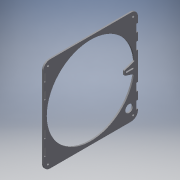
# Autodesk Inventor part: TrayPanelD_180mm
Saved by Autodesk Inventor 2017 (Build 210142000, 142)
## iProperties
Created: 2019-06-22
Part Number: TrayPanelD_180mm
Material: Generic
Document SubType Name: Modeling
Designer: DDeGo
Density: 1 g/cm^3
Appearance: Default
Author: DDeGo
Autodesk Inventor part; units mm, degrees
ref_plane "YZ Plane" through (0, 0, 0) normal (1, 0, 0) x (0, 1, 0)
ref_plane "XZ Plane" through (0, 0, 0) normal (0, 1, 0) x (-1, 0, 0)
ref_plane "XY Plane" through (0, 0, 0) normal (0, 0, 1) x (1, 0, 0)
sketch "Sketch1" plane through (0, 0, 0) normal (1, 0, 0) x (0, 1, 0)
  circle A0 centre (-4, -4) radius 2
  circle A1 centre (78.5, 78.5) radius 85
  circle A2 centre (161, -4) radius 2
  circle A3 centre (-4, 161) radius 2
  circle A4 centre (161, 161) radius 2
  line L0 (157, 170) -> (0, 170)
  arc A5 (0, 170) -> (-13, 157) centre (0, 157) ccw
  line L1 (-13, 157) -> (-13, 0)
  arc A6 (-13, 0) -> (0, -13) centre (0, 0) ccw
  line L2 (0, -13) -> (157, -13)
  arc A7 (157, -13) -> (170, 0) centre (157, 0) ccw
  line L3 (170, 0) -> (170, 157)
  arc A8 (170, 157) -> (157, 170) centre (157, 157) ccw
  line L4 (-4, 161) -> (161, 161) construction
  line L5 (161, 161) -> (161, -4) construction
  line L6 (161, -4) -> (-4, -4) construction
  line L7 (-4, -4) -> (-4, 161) construction
  line L8 (-4, 161) -> (161, -4) construction
  line L9 (-13, 78.5) -> (78.5, 78.5) construction
  line L10 (78.5, 78.5) -> (170, 78.5) construction
  dimension "d10" = 183
  dimension "d11" = 183
  dimension "d12" = 165
  dimension "d13" = 165
  dimension "d15" = 13
  dimension "d16" = 4
  dimension "d17" = 170
  constraints: 22 end point, 9 centre point, 8 point on circle, 8 tangent, 6 equal radius, 3 horizontal, 3 midpoint, 3 perpendicular, 1 coincident, 1 collinear, 1 vertical
  measures "d10" distance between parallel lines of L3 L1
  measures "d11" distance between parallel lines of L0 L2
  measures "d12" distance between parallel lines of L5 L7
  measures "d13" distance of L4.end L5.end
  measures "d15" radius of A5
  measures "d16" diameter of A4
  measures "d17" diameter of A1
extrude "Extrusion1" add sketch "Sketch1" along normal blind 2.75
sketch "Sketch2" plane through (2.75, 0, 0) normal (1, 0, 0) x (0, 0, -1)
  line L0 (0, 170) -> (-157, 170) projected
  line L1 (-146.1, 170) -> (-131.1, 170)
  line L2 (-131.1, 170) -> (-131.1, 166.5)
  line L3 (-131.1, 166.5) -> (-146.1, 166.5)
  line L4 (-146.1, 166.5) -> (-146.1, 170)
  line L5 (-116.1, 170) -> (-101.1, 170)
  line L6 (-101.1, 170) -> (-101.1, 166.5)
  line L7 (-101.1, 166.5) -> (-116.1, 166.5)
  line L8 (-116.1, 166.5) -> (-116.1, 170)
  line L9 (-47.1, 170) -> (-32.1, 170)
  line L10 (-32.1, 170) -> (-32.1, 166.5)
  line L11 (-32.1, 166.5) -> (-47.1, 166.5)
  line L12 (-47.1, 166.5) -> (-47.1, 170)
  line L13 (-2.1, 170) -> (-17.1, 170)
  line L14 (-17.1, 170) -> (-17.1, 166.5)
  line L15 (-17.1, 166.5) -> (-2.1, 166.5)
  line L16 (-2.1, 166.5) -> (-2.1, 170)
  circle A0 centre (-161, 161) radius 2 projected
  point P0 (0, 0)
  dimension "d2" = 15
  dimension "d3" = 30
  dimension "d4" = 69
  dimension "d5" = 30
  dimension "d6" = 3.5
  dimension "d7" = 14.9
  constraints: 32 end point, 8 parallel, 7 point on line, 4 horizontal, 4 perpendicular, 3 collinear
  measures "d2" distance of L2.end L3.end
  measures "d3" distance between parallel lines of L6 L2
  measures "d4" distance between parallel lines of L10 L6
  measures "d5" distance between parallel lines of L16 L10
  measures "d6" distance of L15.end L13.start
  measures "d7" distance from line of L4 A0.centre
extrude "Extrusion2" cut sketch "Sketch2" against normal blind 10 contours L16 L15 L14 L0 | L10 L11 L12 L0 | L6 L7 L8 L0 | L2 L3 L4 L0
sketch "Sketch3" plane through (2.75, 0, 0) normal (1, 0, 0) x (0, 0, -1)
  line L0 (-56.4, -11.425) -> (-41.4, -11.425)
  line L1 (-41.4, -11.425) -> (-41.4, -8.675)
  line L2 (-41.4, -8.675) -> (-56.4, -8.675)
  line L3 (-56.4, -8.675) -> (-56.4, -11.425)
  line L4 (-26.4, -11.425) -> (-11.4, -11.425)
  line L5 (-11.4, -11.425) -> (-11.4, -8.675)
  line L6 (-11.4, -8.675) -> (-26.4, -8.675)
  line L7 (-26.4, -8.675) -> (-26.4, -11.425)
  line L8 (-106.4, -11.425) -> (-121.4, -11.425)
  line L9 (-121.4, -11.425) -> (-121.4, -8.675)
  line L10 (-121.4, -8.675) -> (-106.4, -8.675)
  line L11 (-106.4, -8.675) -> (-106.4, -11.425)
  line L12 (-136.4, -11.425) -> (-151.4, -11.425)
  line L13 (-151.4, -11.425) -> (-151.4, -8.675)
  line L14 (-151.4, -8.675) -> (-136.4, -8.675)
  line L15 (-136.4, -8.675) -> (-136.4, -11.425)
  line L16 (-157, -13) -> (0, -13) projected
  circle A0 centre (-161, -4) radius 2 projected
  point P0 (0, 0)
  dimension "d18" = 1.575
  dimension "d19" = 30
  dimension "d20" = 65
  dimension "d21" = 30
  dimension "d22" = 2.75
  dimension "d23" = 9.6
  dimension "d26" = 15
  constraints: 32 end point, 8 parallel, 6 point on line, 4 horizontal, 4 perpendicular, 3 collinear
  measures "d18" distance between parallel lines of L16 L12
  measures "d19" distance between parallel lines of L11 L15
  measures "d20" distance between parallel lines of L1 L11
  measures "d21" distance between parallel lines of L5 L1
  measures "d22" distance of L4.end L5.end
  measures "d23" distance from line of A0.centre L13
  measures "d26" distance of L12.start L12.end
extrude "Extrusion3" cut sketch "Sketch3" against normal blind 10 contours L3 L2 L1 L0 | L7 L6 L5 L4 | L8 L9 L10 L11 | L12 L13 L14 L15
sketch "Sketch4" plane through (2.75, 0, 0) normal (1, 0, 0) x (0, 0, -1)
  line L0 (-75.85, 147) -> (-73.1, 147)
  line L1 (-73.1, 147) -> (-73.1, 162)
  line L2 (-73.1, 162) -> (-75.85, 162)
  line L3 (-75.85, 162) -> (-75.85, 147)
  line L4 (-78.85, 144) -> (-70.1, 144)
  line L5 (-70.1, 144) -> (-63.1, 165)
  line L6 (-63.1, 165) -> (-85.85, 165)
  line L7 (-85.85, 165) -> (-78.85, 144)
  line L8 (-47.1, 170) -> (-101.1, 170) projected
  line L9 (-47.1, 166.5) -> (-47.1, 170) projected
  point P0 (0, 0)
  dimension "d27" = 8
  dimension "d28" = 26
  dimension "d29" = 2.75
  dimension "d30" = 15
  dimension "d31" = 3
  dimension "d32" = 3
  dimension "d33" = 3
  dimension "d34" = 10
  dimension "d35" = 10
  dimension "d36" = 5
  constraints: 16 end point, 3 parallel, 2 horizontal, 1 perpendicular
  measures "d27" distance between parallel lines of L8 L2
  measures "d28" distance between parallel lines of L9 L1
  measures "d29" distance of L1.end L2.end
  measures "d30" distance of L0.end L1.end
  measures "d31" distance between parallel lines of L4 L0
  measures "d32" distance from line of L4.start L3
  measures "d33" distance from line of L4.end L1
  measures "d34" distance from line of L5.end L1
  measures "d35" distance from line of L6.end L3
  measures "d36" distance between parallel lines of L8 L6
extrude "Extrusion4" add sketch "Sketch4" against normal up to surface (2.75 mm away)
fillet "Fillet1" radius 2 4 edges at (1.375, 144, 78.85) (1.375, 144, 70.1) (1.375, 163.2307, 85.2602) (1.375, 162.2566, 64.0145)
sketch "Sketch5" plane through (2.75, 0, 0) normal (1, 0, 0) x (0, 0, -1)
  circle A0 centre (-11, 153) radius 7.5
  circle A1 centre (4, 161) radius 2 projected
  point P0 (0, 0)
  dimension "d40" = 15
  dimension "d41" = 15
  dimension "d42" = 8
  constraints: 1 centre point
  measures "d40" diameter of A0
  measures "d41" horizontal distance of A0.centre A1.centre
  measures "d42" vertical distance of A0.centre A1.centre
extrude "Extrusion5" cut sketch "Sketch5" against normal blind 10 contours A0
body "Solid1"
